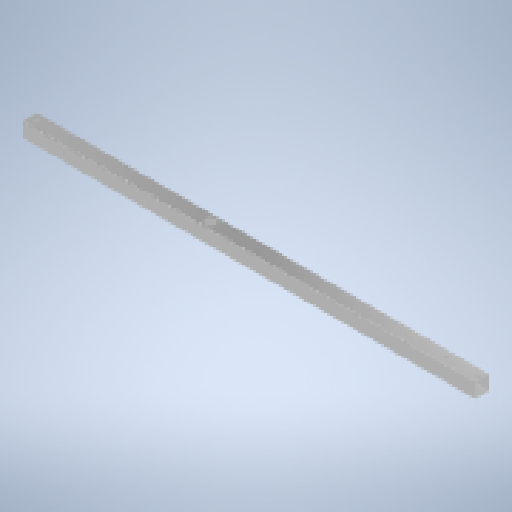
# Autodesk Inventor part: Längs_Traverse_hinten
Saved by Autodesk Inventor 2024.4 (Build 284460000, 460)
## iProperties
Created: 2026-01-06
Part Number: Längs_Traverse_hinten
Material: Aluminium 6061
Description: Längs_Traverse_hinten
Document SubType Name: Modeling
Designer: julia
Mass: 1013.68 g
Surface Area: 3744.88 cm^2
Volume: 375.439 cm^3
Density: 2.7 g/cm^3
Appearance: Aluminium - flach
DocNumber: Längs_Traverse_hinten.ipt
Folder: I60-Konstruktion\I60-Gruppe-7\Gestell\
VDS_Category: Konstruktion
Masse[kg]: 0,378 kg
Autodesk Inventor part; units mm, degrees
ref_plane "YZ Plane" through (0, 0, 0) normal (1, 0, 0) x (0, 1, 0)
ref_plane "XZ Plane" through (0, 0, 0) normal (0, 1, 0) x (-1, 0, 0)
ref_plane "XY Plane" through (0, 0, 0) normal (0, 0, 1) x (1, 0, 0)
sketch "Skizze1" plane through (0, 0, 0) normal (1, 0, 0) x (0, 1, 0)
  line L0 (-20, 20) -> (20, 20)
  line L1 (20, 20) -> (20, -20)
  line L2 (20, -20) -> (-20, -20)
  line L3 (-20, -20) -> (-20, 20)
  line L4 (-20, 20) -> (20, -20) construction
  line L5 (20, 20) -> (-20, -20) construction
  line L6 (-18, 18) -> (18, 18)
  line L7 (18, 18) -> (18, -18)
  line L8 (18, -18) -> (-18, -18)
  line L9 (-18, -18) -> (-18, 18)
  line L10 (-18, 18) -> (18, -18) construction
  line L11 (18, 18) -> (-18, -18) construction
  point P0 (0, 0)
  dimension "d0" = 40
  dimension "d1" = 40
  dimension "d2" = 36
  dimension "d3" = 36
  constraints: 24 end point, 4 midpoint, 4 parallel, 2 horizontal, 2 perpendicular
  measures "d0" distance of L1.end L2.end
  measures "d1" distance of L0.end L1.end
  measures "d2" distance of L7.end L8.end
  measures "d3" distance of L6.end L7.end
extrude "Extrusion1" add sketch "Skizze1" along normal blind 1250
sketch "Skizze2" plane through (0, -20, 20) normal (0, 0, 1) x (1, 0, 0)
  circle A0 centre (20, 20) radius 5.25
  line L0 (1250, 2) -> (1250, 38) projected
  circle A1 centre (1150, 20) radius 5.25
  point P0 (0, 20)
  dimension "d7" = 10.5
  dimension "d11" = 10.5
  constraints: 2 centre point
  measures "d7" diameter of A0
  measures "d11" diameter of A1
extrude "Extrusion2" cut sketch "Skizze2" against normal blind 1250
sketch "Skizze3" plane through (0, 20, 20) normal (0, 1, 0) x (1, 0, 0)
  line L0 (0, 20) -> (110, 20)
  circle A0 centre (110, 20) radius 3.2
  dimension "d14" = 110
  dimension "d15" = 6.4
  constraints: 2 end point, 1 centre point, 1 coincident, 1 horizontal
  measures "d14" distance of L0.start L0.end
  measures "d15" diameter of A0
extrude "Extrusion3" cut sketch "Skizze3" against normal blind 5
sketch "Skizze4" plane through (0, -20, -20) normal (0, -1, 0) x (1, 0, 0)
  circle A0 centre (110, 20) radius 3.2 projected
  line L0 (0, 20) -> (110, 20)
  circle A1 centre (110, 20) radius 5.5
  dimension "d18" = 110
  dimension "d19" = 11
  constraints: 2 end point, 1 centre point, 1 coincident, 1 horizontal
  measures "d18" distance of L0.start L0.end
  measures "d19" diameter of A1
extrude "Extrusion4" cut sketch "Skizze4" against normal blind 5 contours A0 | A1
fillet "Rundung1" radius 1 4 edges at (625, 20, -20) (625, -20, -20) (625, -20, 20) (625, 20, 20)
fillet "Rundung2" radius 0.5 4 edges at (625, -18, 18) (625, -18, -18) (625, 18, -18) (625, 18, 18)
sketch "Skizze6" plane through (0, -19, -20) normal (0, 0, -1) x (-1, 0, 0)
  line L0 (0, 19) -> (-500, 19)
  circle A0 centre (-500, 19) radius 14
  dimension "d28" = 500
  dimension "d29" = 28
  constraints: 2 end point, 1 centre point, 1 coincident, 1 horizontal
  measures "d28" distance of L0.start L0.end
  measures "d29" diameter of A0
extrude "Extrusion6" cut sketch "Skizze6" against normal blind 40
sketch "Skizze7" plane through (0, -19, 20) normal (0, 0, 1) x (1, 0, 0)
  line L0 (1250, 0) -> (1250, 38) projected
  line L1 (1250, 19) -> (1240, 19)
  circle A0 centre (1240, 19) radius 5.25
  point P0 (0, 19)
  dimension "d32" = 10
  dimension "d33" = 10.5
  constraints: 2 end point, 1 centre point, 1 coincident, 1 horizontal, 1 midpoint
  measures "d32" distance of L1.start L1.end
  measures "d33" diameter of A0
extrude "Extrusion7" cut sketch "Skizze7" against normal through all
